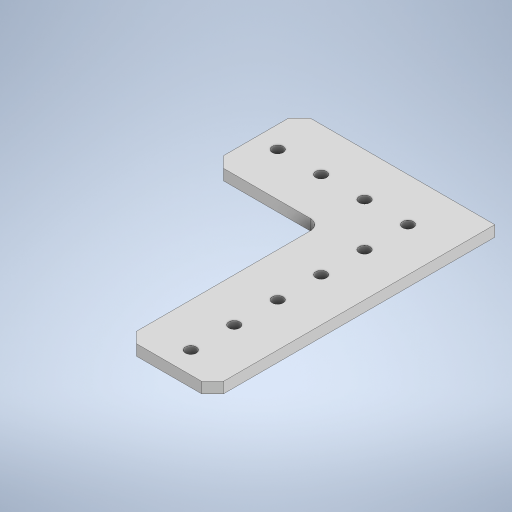
# Autodesk Inventor part: L-Bracket (4x6)
Saved by Autodesk Inventor 2023 (Build 270158030, 158C)
## iProperties
Created: 2022-07-21
Part Number: L-Bracket (4x6)
Material: Generic
Document SubType Name: Modeling
Designer: rm0990889
Density: 1 g/cm^3
Appearance: Default
Author: rm0990889
Autodesk Inventor part; units mm, degrees
ref_plane "YZ Plane" through (0, 0, 0) normal (1, 0, 0) x (0, 1, 0)
ref_plane "XZ Plane" through (0, 0, 0) normal (0, 1, 0) x (-1, 0, 0)
ref_plane "XY Plane" through (0, 0, 0) normal (0, 0, 1) x (1, 0, 0)
sketch "Sketch1" plane through (0, 0, 0) normal (0, 1, 0) x (-1, 0, 0)
  line L0 (4.9142, 0) -> (0, 0)
  line L1 (0, 0) -> (0, 7.2679)
  circle A0 centre (12.7, 12.7) radius 1.5875
  circle A1 centre (25.4, 12.7) radius 1.5875
  circle A2 centre (38.1, 12.7) radius 1.5875
  circle A3 centre (50.8, 12.7) radius 1.5875
  circle A4 centre (12.7, 25.4) radius 1.5875
  circle A5 centre (12.7, 38.1) radius 1.5875
  circle A6 centre (12.7, 50.8) radius 1.5875
  circle A7 centre (12.7, 63.5) radius 1.5875
  circle A8 centre (12.7, 76.2) radius 1.5875
  line L2 (0, 7.2679) -> (0, 79.375)
  line L3 (3.175, 82.55) -> (22.225, 82.55)
  line L4 (25.4, 79.375) -> (25.4, 28.575)
  line L5 (28.575, 25.4) -> (53.975, 25.4)
  line L6 (57.15, 22.225) -> (57.15, 3.175)
  line L7 (53.975, 0) -> (4.9142, 0)
  line L8 (57.15, 22.225) -> (53.975, 25.4)
  line L9 (57.15, 3.175) -> (53.975, 0)
  line L10 (3.175, 82.55) -> (0, 79.375)
  line L11 (22.225, 82.55) -> (25.4, 79.375)
  arc A9 (25.4, 28.575) -> (28.575, 25.4) centre (28.575, 28.575) ccw
  point P0 (2.4571, 0)
  point P1 (0, 82.55)
  point P2 (25.4, 82.55)
  point P3 (25.4, 25.4)
  point P4 (57.15, 25.4)
  point P5 (57.15, 0)
  point P6 (57.15, 12.7)
  dimension "d0" = 3.175
  dimension "d1" = 12.7
  dimension "d2" = 12.7
  dimension "d5" = 12.7
  dimension "d12" = 12.7
  dimension "d17" = 25.4
  dimension "d18" = 6.35
  dimension "d19" = 12.7
  dimension "d20" = 6.35
  dimension "d21" = 3.175
  dimension "d22" = 3.175
  dimension "d23" = 3.175
  dimension "d24" = 3.175
  dimension "d25" = 3.175
  dimension "d26" = 3.175
  dimension "d27" = 3.175
  dimension "d28" = 3.175
  dimension "d29" = 3.175
  constraints: 24 end point, 10 centre point, 10 point on line, 5 perpendicular, 3 horizontal, 2 midpoint, 2 point on circle, 2 tangent, 2 vertical, 16 other
  measures "d0" diameter of A0
  measures "d1" vertical distance of point (2.457, 0) A0.centre
  measures "d2" distance from line of L1 A0.centre
  measures "d5" distance of A0.centre A1.centre
  measures "d12" distance of A0.centre A4.centre
  measures "d17" distance of point (0, 82.55) point (25.4, 82.55)
  measures "d18" distance from line of A8.centre L3
  measures "d19" distance of A1.centre point (25.4, 25.4)
  measures "d20" distance of A3.centre point (57.15, 12.7)
  measures "d21" distance of L6.start point (57.15, 25.4)
  measures "d22" distance of L5.end point (57.15, 25.4)
  measures "d23" distance of L6.end point (57.15, 0)
  measures "d24" distance of L7.start point (57.15, 0)
  measures "d25" distance of L3.start point (0, 82.55)
  measures "d26" distance of L2.end point (0, 82.55)
  measures "d27" distance of L3.end point (25.4, 82.55)
  measures "d28" distance of L4.start point (25.4, 82.55)
  measures "d29" radius of A9
extrude "Extrusion1" add sketch "Sketch1" along normal blind 3.175
equation "\"d22\" = d21"
equation "\"d23\" = d21"
equation "\"d24\" = d23"
equation "\"d26\" = d25"
equation "\"d27\" = d25"
equation "\"d28\" = d27"
body "Solid1"
